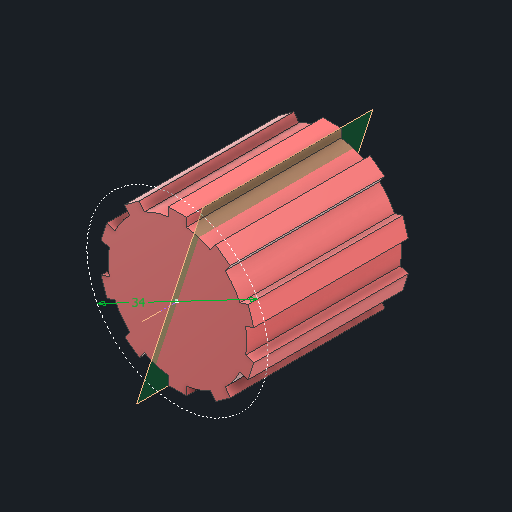
# Autodesk Inventor part: felga_CPY
Saved by Autodesk Inventor 2024 (Build 280153000, 153)
## iProperties
Created: 2024-05-21
Part Number: felga_CPY
Material: Generic
Document SubType Name: Modeling
Designer: Adam
Density: 1 g/cm^3
Appearance: Default
Author: Adam
Autodesk Inventor part; units mm, degrees
ref_plane "YZ Plane" through (0, 0, 0) normal (1, 0, 0) x (0, 1, 0)
ref_plane "XZ Plane" through (0, 0, 0) normal (0, 1, 0) x (-1, 0, 0)
sketch "Sketch1" plane through (0, 0, 0) normal (0, 0, 1) x (1, 0, 0)
  circle A0 centre (0, 0) radius 17 construction
  circle A1 centre (0, 0) radius 8.5
  line L0 (-1.727, 14.5) -> (1.69, 14.5)
  line L1 (1.69, 14.5) -> (1.69, 12.8897)
  line L2 (-1.727, 12.8848) -> (-1.727, 14.5)
  line L3 (-7.1557, 12.7241) -> (-6.2091, 11.4213)
  line L4 (-9.92, 10.7157) -> (-7.1557, 12.7241)
  line L5 (-8.9706, 9.4089) -> (-9.92, 10.7157)
  line L6 (-13.2681, 6.088) -> (-11.7366, 5.5904)
  line L7 (-14.324, 2.8383) -> (-13.2681, 6.088)
  line L8 (-12.7878, 2.3392) -> (-14.324, 2.8383)
  line L9 (-14.3126, -2.8735) -> (-12.7811, -2.3759)
  line L10 (-13.2567, -6.1232) -> (-14.3126, -2.8735)
  line L11 (-11.7205, -5.624) -> (-13.2567, -6.1232)
  line L12 (-9.8901, -10.7374) -> (-8.9436, -9.4346)
  line L13 (-7.1258, -12.7458) -> (-9.8901, -10.7374)
  line L14 (-6.1764, -11.4391) -> (-7.1258, -12.7458)
  line L15 (-1.69, -14.5) -> (-1.69, -12.8897)
  line L16 (1.727, -14.5) -> (-1.69, -14.5)
  line L17 (1.727, -12.8848) -> (1.727, -14.5)
  line L18 (7.1557, -12.7241) -> (6.2091, -11.4213)
  line L19 (9.92, -10.7157) -> (7.1557, -12.7241)
  line L20 (8.9706, -9.4089) -> (9.92, -10.7157)
  line L21 (13.2681, -6.088) -> (11.7366, -5.5904)
  line L22 (14.324, -2.8383) -> (13.2681, -6.088)
  line L23 (12.7878, -2.3392) -> (14.324, -2.8383)
  line L24 (14.3126, 2.8735) -> (12.7811, 2.3759)
  line L25 (13.2567, 6.1232) -> (14.3126, 2.8735)
  line L26 (11.7205, 5.624) -> (13.2567, 6.1232)
  line L27 (9.8901, 10.7374) -> (8.9436, 9.4346)
  line L28 (7.1258, 12.7458) -> (9.8901, 10.7374)
  line L29 (6.1764, 11.4391) -> (7.1258, 12.7458)
  arc A2 (-1.727, 12.8848) -> (-6.2091, 11.4213) centre (0, 0) ccw construction
  arc A3 (-1.727, 12.8848) -> (-6.2091, 11.4213) centre (0, 0) ccw
  arc A4 (-8.9706, 9.4089) -> (-11.7366, 5.5904) centre (0, 0) ccw
  arc A5 (-8.9706, 9.4089) -> (-11.7366, 5.5904) centre (0, 0) ccw construction
  arc A6 (-12.7878, 2.3392) -> (-12.7811, -2.3759) centre (0, 0) ccw
  arc A7 (-12.7878, 2.3392) -> (-12.7811, -2.3759) centre (0, 0) ccw construction
  arc A8 (-11.7205, -5.624) -> (-8.9436, -9.4346) centre (0, 0) ccw
  arc A9 (-11.7205, -5.624) -> (-8.9436, -9.4346) centre (0, 0) ccw construction
  arc A10 (6.1764, 11.4391) -> (1.69, 12.8897) centre (0, 0) ccw construction
  arc A11 (6.1764, 11.4391) -> (1.69, 12.8897) centre (0, 0) ccw
  arc A12 (12.7878, -2.3392) -> (12.7811, 2.3759) centre (0, 0) ccw
  arc A13 (12.7878, -2.3392) -> (12.7811, 2.3759) centre (0, 0) ccw construction
  arc A14 (8.9706, -9.4089) -> (11.7366, -5.5904) centre (0, 0) ccw
  arc A15 (8.9706, -9.4089) -> (11.7366, -5.5904) centre (0, 0) ccw construction
  arc A16 (-6.1764, -11.4391) -> (-1.69, -12.8897) centre (0, 0) ccw
  arc A17 (1.727, -12.8848) -> (6.2091, -11.4213) centre (0, 0) ccw
  arc A18 (-6.1764, -11.4391) -> (-1.69, -12.8897) centre (0, 0) ccw construction
  arc A19 (1.727, -12.8848) -> (6.2091, -11.4213) centre (0, 0) ccw construction
  arc A20 (11.7205, 5.624) -> (8.9436, 9.4346) centre (0, 0) ccw
  dimension "d5" = 360
  dimension "d14" = 6
  dimension "d15" = 13
  dimension "d16" = 34
  dimension "d17" = 17
  constraints: 60 end point, 38 point on circle, 21 centre point, 5 coincident, 1 horizontal, 1 parallel, 1 perpendicular, 71 other
  measures "d14" distance edge to line of A1 L0
  measures "d15" radius of A2
  measures "d16" diameter of A0
  measures "d17" diameter of A1
extrude "Extrusion1" add sketch "Sketch1" along normal blind 29
sketch "Sketch2" plane through (0, 0, 29) normal (0, 0, 1) x (1, 0, 0)
  line L0 (-6.2091, 11.4213) -> (-7.1557, 12.7241) projected
  line L1 (-7.1557, 12.7241) -> (-9.92, 10.7157) projected
  line L2 (-9.92, 10.7157) -> (-8.9706, 9.4089) projected
  arc A0 (-8.9706, 9.4089) -> (-11.7366, 5.5904) centre (0, 0) ccw projected
  line L3 (-11.7366, 5.5904) -> (-13.2681, 6.088) projected
  line L4 (-13.2681, 6.088) -> (-14.324, 2.8383) projected
  line L5 (-14.324, 2.8383) -> (-12.7878, 2.3392) projected
  arc A1 (-12.7878, 2.3392) -> (-12.7811, -2.3759) centre (0, 0) ccw projected
  line L6 (-12.7811, -2.3759) -> (-14.3126, -2.8735) projected
  line L7 (-14.3126, -2.8735) -> (-13.2567, -6.1232) projected
  line L8 (-13.2567, -6.1232) -> (-11.7205, -5.624) projected
  arc A2 (-11.7205, -5.624) -> (-8.9436, -9.4346) centre (0, 0) ccw projected
  line L9 (-8.9436, -9.4346) -> (-9.8901, -10.7374) projected
  line L10 (-9.8901, -10.7374) -> (-7.1258, -12.7458) projected
  line L11 (-7.1258, -12.7458) -> (-6.1764, -11.4391) projected
  arc A3 (-6.1764, -11.4391) -> (-1.69, -12.8897) centre (0, 0) ccw projected
  line L12 (-1.69, -12.8897) -> (-1.69, -14.5) projected
  line L13 (-1.69, -14.5) -> (1.727, -14.5) projected
  line L14 (1.727, -14.5) -> (1.727, -12.8848) projected
  arc A4 (1.727, -12.8848) -> (6.2091, -11.4213) centre (0, 0) ccw projected
  line L15 (6.2091, -11.4213) -> (7.1557, -12.7241) projected
  line L16 (7.1557, -12.7241) -> (9.92, -10.7157) projected
  line L17 (9.92, -10.7157) -> (8.9706, -9.4089) projected
  arc A5 (8.9706, -9.4089) -> (11.7366, -5.5904) centre (0, 0) ccw projected
  line L18 (11.7366, -5.5904) -> (13.2681, -6.088) projected
  line L19 (13.2681, -6.088) -> (14.324, -2.8383) projected
  line L20 (14.324, -2.8383) -> (12.7878, -2.3392) projected
  arc A6 (12.7878, -2.3392) -> (12.7811, 2.3759) centre (0, 0) ccw projected
  line L21 (12.7811, 2.3759) -> (14.3126, 2.8735) projected
  line L22 (14.3126, 2.8735) -> (13.2567, 6.1232) projected
  line L23 (13.2567, 6.1232) -> (11.7205, 5.624) projected
  arc A7 (11.7205, 5.624) -> (8.9436, 9.4346) centre (0, 0) ccw projected
  line L24 (8.9436, 9.4346) -> (9.8901, 10.7374) projected
  line L25 (9.8901, 10.7374) -> (7.1258, 12.7458) projected
  line L26 (7.1258, 12.7458) -> (6.1764, 11.4391) projected
  arc A8 (6.1764, 11.4391) -> (1.69, 12.8897) centre (0, 0) ccw projected
  line L27 (1.69, 12.8897) -> (1.69, 14.5) projected
  line L28 (1.69, 14.5) -> (-1.727, 14.5) projected
  line L29 (-1.727, 14.5) -> (-1.727, 12.8848) projected
  arc A9 (-1.727, 12.8848) -> (-6.2091, 11.4213) centre (0, 0) ccw projected
  circle A10 centre (0, 0) radius 8.5 projected
  circle A11 centre (0, 0) radius 8.5
  constraints: 1 centre point, 1 coincident, 1 concentric
extrude "Extrusion2" add sketch "Sketch2" against normal blind 11 contours A10
sketch "Sketch3" plane through (0, 0, 18) normal (0, 0, -1) x (-1, 0, 0)
  arc A0 (1.3217, 0.7094) -> (0.5581, -1.3923) centre (0, 0) ccw
  line L0 (0.5581, -1.3923) -> (1.3217, 0.7094)
  circle A1 centre (0, 0) radius 2.5
  point P0 (0, 0)
  dimension "d11" = 5
  constraints: 2 centre point, 2 end point, 2 point on circle, 1 coincident, 1 other
  measures "d11" diameter of A1
extrude "Extrusion3" add sketch "Sketch3" along normal blind 9
ref_plane "Work Plane1" through (-0.5337, -1.6424, 0) normal (-0.9511, 0.309, 0) x (0, 0, 1)
sketch "Sketch4" plane through (-0.5337, -1.6424, 0) normal (-0.9511, 0.309, 0) x (0, 0, 1)
  line L0 (31.9338, 1.727) -> (-3.3978, 1.727) construction
  point P0 (0, 1.727)
  constraints: 2 end point, 1 horizontal
ref_plane "Work Plane2" through (0, 0, 29) normal (0, 0, 1) x (1, 0, 0)
sketch "Sketch5" plane through (0, 0, 29) normal (0, 0, 1) x (1, 0, 0)
  circle A0 centre (0, 0) radius 17 construction
  dimension "d19" = 34
  constraints: 1 centre point, 1 coincident
  measures "d19" diameter of A0
body "Solid1"
